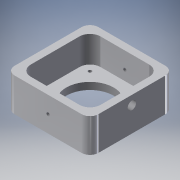
# Autodesk Inventor part: basemotor
Saved by Autodesk Inventor 2016 (Build 200138000, 138)
## iProperties
Created: 2017-12-18
Part Number: basemotor
Material: Generic
Document SubType Name: Modeling
Designer: student
Density: 1 g/cm^3
Appearance: Default
Author: student
Autodesk Inventor part; units mm, degrees
ref_plane "YZ Plane" through (0, 0, 0) normal (1, 0, 0) x (0, 1, 0)
ref_plane "XZ Plane" through (0, 0, 0) normal (0, 1, 0) x (-1, 0, 0)
sketch "Sketch2" plane through (0, 0, 0) normal (0, 1, 0) x (-1, 0, 0)
  line L0 (-31.75, 31.75) -> (31.75, 31.75)
  line L1 (31.75, 31.75) -> (31.75, -31.75)
  line L2 (31.75, -31.75) -> (-31.75, -31.75)
  line L3 (-31.75, -31.75) -> (-31.75, 31.75)
  line L4 (-31.75, 31.75) -> (31.75, -31.75) construction
  line L5 (31.75, 31.75) -> (-31.75, -31.75) construction
  point P0 (0, 0)
  dimension "d3" = 63.5
  dimension "d4" = 63.5
  constraints: 12 end point, 2 midpoint, 2 parallel, 1 horizontal, 1 perpendicular
  measures "d3" distance of L1.end L2.end
  measures "d4" distance of L0.end L1.end
extrude "Extrusion2" add sketch "Sketch2" along normal blind 25.4
fillet "Fillet1" radius 6.35 4 edges at (31.75, 12.7, 31.75) (31.75, 12.7, -31.75) (-31.75, 12.7, -31.75) (-31.75, 12.7, 31.75)
sketch "Sketch3" plane through (0, 25.4, 0) normal (0, 1, 0) x (1, 0, 0)
  arc A0 (-31.75, -25.4) -> (-25.4, -31.75) centre (-25.4, -25.4) ccw projected
  line L0 (-25.4, -31.75) -> (25.4, -31.75) projected
  arc A1 (25.4, -31.75) -> (31.75, -25.4) centre (25.4, -25.4) ccw projected
  line L1 (31.75, -25.4) -> (31.75, 25.4) projected
  arc A2 (31.75, 25.4) -> (25.4, 31.75) centre (25.4, 25.4) ccw projected
  line L2 (25.4, 31.75) -> (-25.4, 31.75) projected
  arc A3 (-25.4, 31.75) -> (-31.75, 25.4) centre (-25.4, 25.4) ccw projected
  line L3 (-31.75, 25.4) -> (-31.75, -25.4) projected
  line L4 (-26.416, 26.416) -> (26.416, 26.416)
  line L5 (26.416, 26.416) -> (26.416, -26.416)
  line L6 (26.416, -26.416) -> (-26.416, -26.416)
  line L7 (-26.416, -26.416) -> (-26.416, 26.416)
  point P0 (0, 0)
  dimension "d8" = 5.334
  constraints: 8 end point, 3 other
  measures "d8" distance between parallel lines of L2 L4
extrude "Extrusion3" cut sketch "Sketch3" against normal blind 20.066 contours L4 L5 L6 L7
ref_plane "Work Plane1" through (0, 25.4, -26.416) normal (-1, 0, 0) x (0, 0, 1)
fillet "Fillet2" radius 7.9375 4 edges at (-26.416, 15.367, 26.416) (-26.416, 15.367, -26.416) (26.416, 15.367, -26.416) (26.416, 15.367, 26.416)
sketch "Sketch6" plane through (-25.4, 0, 31.75) normal (0, 0, 1) x (1, 0, 0)
  line L0 (0, 0) -> (0, 25.4) projected
  line L1 (50.8, 0) -> (0, 0) projected
  line L2 (50.8, 25.4) -> (50.8, 0) projected
  line L3 (0, 25.4) -> (50.8, 25.4) projected
  circle A0 centre (25.4, 12.7) radius 1.27
  point P0 (25.4, 0)
  dimension "d31" = 2.54
  dimension "d32" = 12.7
  dimension "d33" = 25.4
  constraints: 1 centre point
  measures "d31" diameter of A0
  measures "d32" distance from line of L1 A0.centre
  measures "d33" distance from line of L0 A0.centre
hole "Hole3" at (0, 12.7, 31.75) direction (0, 0, -1) diameter 2.54 depth 76.2 tip angle 118
sketch "Sketch8" plane through (0, 0, 0) normal (0, -1, 0) x (1, 0, 0)
  point P0 (0, 0)
sketch "Sketch9" plane through (0, 0, 0) normal (0, -1, 0) x (1, 0, 0)
  line L0 (25.4, 28.575) -> (-15.875, 28.575)
  arc A0 (-15.875, 28.575) -> (-28.575, 15.875) centre (-15.875, 15.875) ccw
  line L1 (-28.575, 15.875) -> (-28.575, -15.875)
  arc A1 (-28.575, -15.875) -> (-15.875, -28.575) centre (-15.875, -15.875) ccw
  line L2 (-15.875, -28.575) -> (25.4, -28.575)
  arc A2 (25.4, -28.575) -> (28.575, -25.4) centre (25.4, -25.4) ccw
  line L3 (28.575, -25.4) -> (28.575, -1.27)
  line L4 (28.575, -1.27) -> (17.9256, -1.27)
  circle A3 centre (0, 0) radius 17.9705
  line L5 (17.9256, 1.27) -> (28.575, 1.27)
  line L6 (28.575, 1.27) -> (28.575, 25.4)
  arc A4 (28.575, 25.4) -> (25.4, 28.575) centre (25.4, 25.4) ccw
  circle A5 centre (-19.685, -19.685) radius 1.27
  circle A6 centre (-19.685, 19.685) radius 1.27
  dimension "d53" = 2.54
  dimension "d54" = 3.81
  dimension "d55" = 3.81
  dimension "d56" = 2.54
  dimension "d57" = 3.81
  dimension "d58" = 3.81
  constraints: 14 end point, 10 point on circle, 7 centre point
  measures "d53" diameter of A5
  measures "d54" horizontal distance of A1.centre A5.centre
  measures "d55" horizontal distance of A1.centre A5.centre
  measures "d56" diameter of A6
  measures "d57" horizontal distance of A0.centre A6.centre
  measures "d58" horizontal distance of A0.centre A6.centre
extrude "Extrusion6" cut sketch "Sketch9" against normal blind 25.4 contours A3 | A5 | A6
sketch "Sketch10" plane through (31.75, 0, 25.4) normal (1, 0, 0) x (0, 0, -1)
  circle A0 centre (25.4, 18.5) radius 3.175
  point P0 (25.4, 0)
  dimension "d61" = 6.35
  constraints: 1 centre point
  measures "d61" diameter of A0
extrude "Extrusion7" cut sketch "Sketch10" against normal blind 6.35
body "Solid2"
